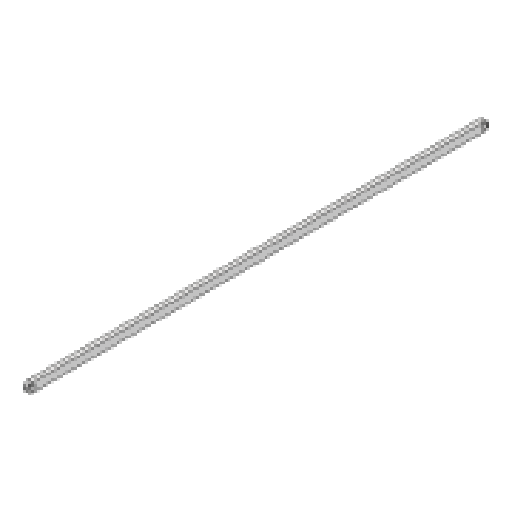
# Autodesk Inventor part: CableManegmentLinkage3
Saved by Autodesk Inventor 2023 (Build 270158000, 158)
## iProperties
Created: 2022-11-13
Part Number: CableManegmentLinkage3
Material: Generic
Document SubType Name: Modeling
Designer: deli
Density: 1 g/cm^3
Appearance: Default
Author: deli
Autodesk Inventor part; units mm, degrees
ref_plane "YZ Plane" through (0, 0, 0) normal (1, 0, 0) x (0, 1, 0)
ref_plane "XZ Plane" through (0, 0, 0) normal (0, 1, 0) x (-1, 0, 0)
ref_plane "XY Plane" through (0, 0, 0) normal (0, 0, 1) x (1, 0, 0)
sketch "Sketch1" plane through (0, 0, 0) normal (1, 0, 0) x (0, 1, 0)
  arc A0 (25.9289, 116.0925) -> (19.9289, 116.0925) centre (22.9289, 116.0925) ccw
  arc A1 (19.9289, -18.9075) -> (25.9289, -18.9075) centre (22.9289, -18.9075) ccw
  circle A2 centre (22.9289, 116.0925) radius 2
  circle A3 centre (22.9289, -18.9075) radius 2
  line L0 (25.9289, 116.0925) -> (25.9289, -18.9075)
  line L1 (19.9289, -18.9075) -> (19.9289, 116.0925)
  point P0 (0, 0)
  dimension "d0" = 4
  dimension "d1" = 6
  dimension "d2" = 135
  constraints: 4 centre point, 4 end point, 4 point on circle, 4 tangent, 2 coincident, 2 equal radius, 1 vertical
  measures "d0" diameter of A2
  measures "d1" diameter of A0
  measures "d2" distance of L0.start L0.end
extrude "Extrusion1" add sketch "Sketch1" along normal blind 3.175
body "Solid1"
